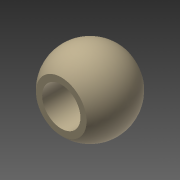
# Autodesk Inventor part: BearingBall
Saved by Autodesk Inventor 2015 (Build 190159000, 159)
## iProperties
Created: 2014-07-13
Part Number: BearingBall
Material: PC/ABS Plastic
Document SubType Name: Modeling
Designer: User
Density: 1.493 g/cm^3
Appearance: Beige
Mass: 0.854825 g
Surface Area: 5.5135 cm^2
Volume: 0.572555 cm^3
Author: User
Autodesk Inventor part; units mm, degrees
ref_plane "YZ Plane" through (0, 0, 0) normal (1, 0, 0) x (0, 1, 0)
ref_plane "XZ Plane" through (0, 0, 0) normal (0, 1, 0) x (-1, 0, 0)
ref_plane "XY Plane" through (0, 0, 0) normal (0, 0, 1) x (1, 0, 0)
sketch "BallDiameter" plane through (0, 0, 0) normal (0, 1, 0) x (-1, 0, 0)
  circle A0 centre (0, 0) radius 6
  line L0 (5.6569, -2) -> (-5.6569, 2)
  dimension "d0" = 12
  constraints: 2 end point, 2 point on circle, 1 centre point, 1 coincident, 1 midpoint
  measures "d0" diameter of A0
revolve "BallFeature" add sketch "BallDiameter" angle 360 about axis through (-5.6569, 0, -2) along (0.942809, 0, 0.3333333) picked at (1.7978, 1.9247) contours A0 L0
sketch "SliceTops" plane through (0, 0, 0) normal (0, 0, 1) x (1, 0, 0)
  line L0 (-11, 0) -> (8.5673, 0) construction
  circle A0 centre (0, 0) radius 6 construction
  line L1 (0, 6) -> (10, 6)
  line L2 (10, 6) -> (10, 4.5)
  line L3 (10, 4.5) -> (0, 4.5)
  line L4 (0, 4.5) -> (0, 6)
  line L5 (0, 6) -> (0, 11) construction
  line L6 (0, 6) -> (-10, 6)
  line L7 (-10, 6) -> (-10, 4.5)
  line L8 (-10, 4.5) -> (0, 4.5)
  line L9 (0, -6) -> (10, -6)
  line L10 (10, -6) -> (10, -4.5)
  line L11 (10, -4.5) -> (0, -4.5)
  line L12 (0, -4.5) -> (0, -6)
  line L13 (0, -6) -> (-10, -6)
  line L14 (-10, -6) -> (-10, -4.5)
  line L15 (-10, -4.5) -> (0, -4.5)
  dimension "d6" = 10
  dimension "d7" = 1.5
  dimension "d8" = 1.4327
  dimension "d9" = 5
  dimension "d10" = 21
  constraints: 32 end point, 8 symmetric about line, 4 parallel, 3 horizontal, 1 perpendicular, 1 vertical alignment, 1 other
  measures "d6" distance of L1.start L1.end
  measures "d7" distance of L1.end L2.end
  measures "d8" distance from line of L0.end L2
  measures "d9" distance from line of L5.end L1
  measures "d10" distance from line of L0.start L2
extrude "SliceTopsFeature" cut sketch "SliceTops" along normal mid plane 10
sketch "Hole" plane through (0, 4.5, 0) normal (0, 1, 0) x (1, 0, 0)
  circle A0 centre (0, 0) radius 3.9686 projected
  circle A1 centre (0, 0) radius 3
  dimension "d13" = 6
  constraints: 1 centre point, 1 coincident
  measures "d13" diameter of A1
hole "HoleFeature" at (0, 4.5, 0) direction (0, -1, 0) diameter 6 end through all
